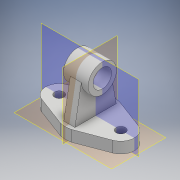
# Autodesk Inventor part: 6.2_DATE11_1
Saved by Autodesk Inventor 2017 (Build 210142000, 142)
## iProperties
Created: 2018-11-01
Part Number: 6.2_DATE11_1
Material: Generic
Document SubType Name: Modeling
Designer: jacob
Density: 1 g/cm^3
Appearance: Default
Author: jacob
Autodesk Inventor part; units mm, degrees
sketch "Sketch1" plane through (0, 0, 0) normal (0, 0, 1) x (1, 0, 0)
  arc A0 (57.763, -20.5849) -> (57.763, 20.5849) centre (50, 0) ccw
  arc A1 (-55.7119, 21.2456) -> (-57.763, -20.5849) centre (-50, 0) ccw
  arc A2 (9, 38.9744) -> (-9, 38.9744) centre (0, 0) ccw
  line L0 (-9, 38.9744) -> (-55.7119, 21.2456)
  line L1 (9, 38.9744) -> (57.763, 20.5849)
  arc A3 (-9, -38.9744) -> (9, -38.9744) centre (0, 0) ccw
  line L2 (-57.763, -20.5849) -> (-9, -38.9744)
  line L3 (9, -38.9744) -> (57.763, -20.5849)
  circle A4 centre (-50, 0) radius 7.5
  circle A5 centre (50, 0) radius 7.5
  dimension "d1" = 50
  dimension "d2" = 100
  dimension "d3" = 44
  dimension "d4" = 44
  dimension "d10" = 40
  dimension "d11" = 18
  dimension "d12" = 9
  dimension "d13" = 0
  dimension "d14" = 138.554
  dimension "d15" = 39.6431
  dimension "d16" = 40
  dimension "d17" = 18
  dimension "d18" = 9
  dimension "d19" = 15
  dimension "d20" = 15
  constraints: 8 end point, 8 point on circle, 6 centre point, 4 coincident, 3 tangent
  measures "d1" distance of point (0, 0) A1.centre
  measures "d2" distance of A0.centre A1.centre
  measures "d3" diameter of A1
  measures "d4" diameter of A0
  measures "d10" radius of A2
  measures "d11" distance of L1.start L0.start
  measures "d12" horizontal distance of point (0, 0) L0.start
  measures "d13" vertical distance of point (0, 0) A0.centre
  measures "d14" angle of L0 L1
  measures "d15" distance from line of point (0, 0) L1
  measures "d16" radius of A3
  measures "d17" distance of L3.start L2.end
  measures "d18" horizontal distance of point (0, 0) L2.end
  measures "d19" diameter of A4
  measures "d20" diameter of A5
extrude "Base" add sketch "Sketch1" along normal blind 18
sketch "Sketch2" plane through (0, 0, 0) normal (1, 0, 0) x (0, 1, 0)
  line L0 (-20.5849, 0) -> (20.5849, 0) projected
  line L1 (20.5849, 0) -> (20.5849, 18) projected
  line L2 (-20.5849, 18) -> (-20.5849, 18) projected
  line L3 (-20.5849, 0) -> (-20.5849, 18) projected
  line L4 (-20.5849, 18) -> (-20.5849, 18) projected
  line L5 (-33.5, 18) -> (33.5, 18)
  line L6 (33.5, 18) -> (23, 76)
  line L7 (23, 76) -> (-23, 76)
  line L8 (-23, 76) -> (-33.5, 18)
  point P0 (0, 0)
  dimension "d23" = 67
  dimension "d24" = 58
  dimension "d25" = 0
  dimension "d26" = 23
  dimension "d27" = 33.5
  dimension "d28" = 46
  constraints: 8 end point, 1 horizontal, 1 parallel
  measures "d23" distance of L5.start L5.end
  measures "d24" distance between parallel lines of L7 L5
  measures "d25" distance between parallel lines of L2 L5
  measures "d26" horizontal distance of point (0, 0) L6.end
  measures "d27" horizontal distance of L5.end point (0, 0)
  measures "d28" distance of L6.end L7.end
extrude "Leg" add sketch "Sketch2" along normal mid plane 18 contours L5 L8 L7 L6
sketch "Sketch3" plane through (0, 0, 0) normal (1, 0, 0) x (0, 1, 0)
  line L0 (-23, 76) -> (23, 76) projected
  circle A0 centre (0, 76) radius 23
  circle A1 centre (0, 76) radius 15
  point P0 (0, 0)
  dimension "d31" = 30
  constraints: 1 centre point, 1 coincident, 1 horizontal alignment, 1 midpoint, 2 other
  measures "d31" diameter of A1
extrude "Circle Ring" add sketch "Sketch3" along normal mid plane 40 contours A1 L0 A0 | L0 A0 A1
extrude "Big Hole Cut" cut sketch "Sketch3" along normal mid plane 40 contours A1 L0 | L0 A1
equation "\"d4\" = d3"
body "Solid1"
